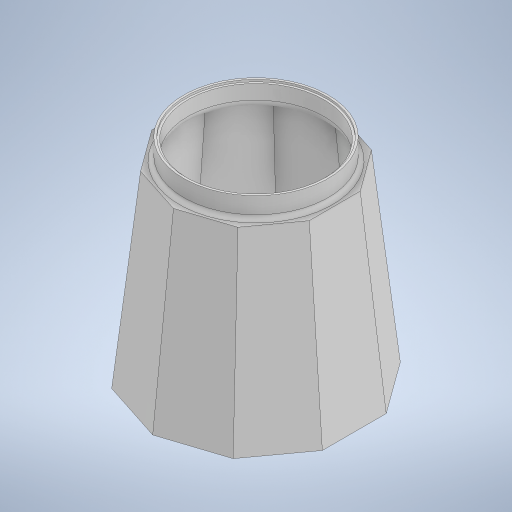
# Autodesk Inventor part: partea_de_jos
Saved by Autodesk Inventor 2024 (Build 280153000, 153)
## iProperties
Created: 2024-01-15
Part Number: partea_de_jos
Material: Generic
Document SubType Name: Modeling
Designer: Sorin
Density: 1 g/cm^3
Appearance: Default
Author: Sorin
Autodesk Inventor part; units mm, degrees
ref_plane "YZ Plane" through (0, 0, 0) normal (1, 0, 0) x (0, 1, 0)
ref_plane "XY Plane" through (0, 0, 0) normal (0, 0, 1) x (1, 0, 0)
sketch "Sketch3" plane through (0, 0, 0) normal (0, 1, 0) x (-1, 0, 0)
  line L0 (0, -50) -> (-29.3893, -40.4508)
  line L1 (-29.3893, -40.4508) -> (-47.5528, -15.4508)
  line L2 (-47.5528, -15.4508) -> (-47.5528, 15.4508)
  line L3 (-47.5528, 15.4508) -> (-29.3893, 40.4508)
  line L4 (-29.3893, 40.4508) -> (0, 50)
  line L5 (0, 50) -> (29.3893, 40.4508)
  line L6 (29.3893, 40.4508) -> (47.5528, 15.4508)
  line L7 (47.5528, 15.4508) -> (47.5528, -15.4508)
  line L8 (47.5528, -15.4508) -> (29.3893, -40.4508)
  line L9 (29.3893, -40.4508) -> (0, -50)
  point P0 (0, 0)
  point P1 (0, 0)
  dimension "d1" = 100
  dimension "d2" = 29.3893
  constraints: 20 end point, 1 coincident, 21 other
  measures "d1" distance of L4.end L0.start
  measures "d2" horizontal distance of L0.start L0.end
ref_plane "Work Plane1" through (0, 90, 0) normal (0, 1, 0) x (-1, 0, 0)
sketch "Sketch4" plane through (0, 90, 0) normal (0, 1, 0) x (-1, 0, 0)
  line L0 (-23.4532, -32.403) -> (-38.02, -12.4291)
  line L1 (-38.02, -12.4291) -> (-38.0645, 12.2923)
  line L2 (-38.0645, 12.2923) -> (-23.5696, 32.3184)
  line L3 (-23.5696, 32.3184) -> (-0.0719, 40)
  line L4 (-0.0719, 40) -> (23.4532, 32.403)
  line L5 (23.4532, 32.403) -> (38.02, 12.4291)
  line L6 (38.02, 12.4291) -> (38.0645, -12.2923)
  line L7 (38.0645, -12.2923) -> (23.5696, -32.3184)
  line L8 (23.5696, -32.3184) -> (0.0719, -40)
  line L9 (0.0719, -40) -> (-23.4532, -32.403)
  point P0 (0, 0)
  point P1 (0, 0)
  dimension "d4" = 80
  dimension "d5" = 23.5251
  constraints: 20 end point, 1 coincident, 21 other
  measures "d4" distance of L3.end L8.end
  measures "d5" horizontal distance of L8.end L0.start
loft "Loft1" add profiles "Sketch3", "Sketch4"
sketch "Sketch6" plane through (-0.0719, 90, -40) normal (0, 1, 0) x (0.9516106, 0, 0.3073066)
  circle A0 centre (12.3607, -38.0423) radius 35
  dimension "d10" = 70
  constraints: 1 centre point, 1 coincident
  measures "d10" diameter of A0
extrude "Extrusion1" add sketch "Sketch6" along normal blind 10
fillet "Fillet1" radius 2 1 edges at (-33.3064, 90, -10.7557)
shell "Shell1" thickness 2 removed faces 1 at (14.8482, 100, -4.0675)
sketch "Sketch7" plane through (0, 100, 0) normal (0, 1, 0) x (1, 0, 0)
  circle A0 centre (0, 0) radius 34
  dimension "d15" = 68
  constraints: 1 centre point, 1 coincident
  measures "d15" diameter of A0
extrude "Extrusion2" cut sketch "Sketch7" against normal blind 1
body "Solid1"
